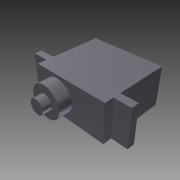
# Autodesk Inventor part: Servo
Saved by Autodesk Inventor 2014 (Build 180170000, 170)
## iProperties
Created: 2014-03-15
Part Number: Servo
Material: Genérico
Document SubType Name: Modeling
Designer: Victor San José Astorga
Density: 1 g/cm^3
Appearance: Acero - Pulido
Author: Victor San José Astorga
Autodesk Inventor part; units mm, degrees
ref_plane "YZ Plane" through (0, 0, 0) normal (1, 0, 0) x (0, 1, 0)
ref_plane "XZ Plane" through (0, 0, 0) normal (0, 1, 0) x (-1, 0, 0)
ref_plane "XY Plane" through (0, 0, 0) normal (0, 0, 1) x (1, 0, 0)
sketch "Boceto1" plane through (0, 0, 0) normal (0, 0, 1) x (1, 0, 0)
  line L0 (0, 0) -> (23, 0)
  line L1 (23, 21) -> (0, 21)
  line L2 (23, 5) -> (28, 5)
  line L3 (28, 5) -> (28, 2.7)
  line L4 (28, 2.7) -> (23, 2.7)
  line L5 (0, 5) -> (-5, 5)
  line L6 (-5, 5) -> (-5, 2.7)
  line L7 (-5, 2.7) -> (0, 2.7)
  line L8 (23, 0) -> (23, 2.7)
  line L9 (23, 5) -> (23, 21)
  line L10 (0, 21) -> (0, 5)
  line L11 (0, 2.7) -> (0, 0)
  dimension "d0" = 23
  dimension "d1" = 21
  dimension "d8" = 5
  dimension "d9" = 2.3
  dimension "d10" = 5
  dimension "d11" = 2.3
  constraints: 24 end point, 10 perpendicular, 6 parallel, 1 horizontal
  measures "d0" distance of L1.end L1.start
  measures "d1" distance of L1.start L0.end
  measures "d8" distance of L2.start L2.end
  measures "d9" distance of L2.end L3.end
  measures "d10" distance of L5.start L5.end
  measures "d11" distance of L5.end L6.end
extrude "Extrusión1" add sketch "Boceto1" along normal blind 12
sketch "Boceto2" plane through (0, 0, 0) normal (0, -1, 0) x (1, 0, 0)
  line L0 (0, 0) -> (0, 12) projected
  circle A0 centre (7.5, 6) radius 5
  dimension "d4" = 10
  dimension "d5" = 7.5
  constraints: 1 centre point
  measures "d4" diameter of A0
  measures "d5" distance from line of L0 A0.centre
extrude "Extrusión2" add sketch "Boceto2" along normal blind 4
sketch "Boceto3" plane through (7.5, -4, 6) normal (0, -1, 0) x (1, 0, 0)
  circle A0 centre (0, 0) radius 5 projected
  circle A1 centre (0, 0) radius 2.33
  point P0 (-7.5, -6)
  dimension "d12" = 4.66
  constraints: 1 centre point, 1 coincident
  measures "d12" diameter of A1
extrude "Extrusión3" add sketch "Boceto3" along normal blind 2.7 contours A1
